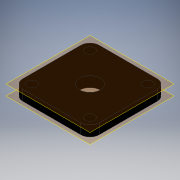
# Autodesk Inventor part: bushing
Saved by Autodesk Inventor 2016 (Build 200138000, 138)
## iProperties
Created: 2015-12-01
Part Number: bushing
Material: Generic
Document SubType Name: Modeling
Designer: Javier
Density: 1 g/cm^3
Appearance: Black
Author: Javier
Autodesk Inventor part; units mm, degrees
ref_plane "YZ Plane" through (0, 0, 0) normal (1, 0, 0) x (0, 1, 0)
ref_plane "XY Plane" through (0, 0, 0) normal (0, 0, 1) x (1, 0, 0)
sketch "Sketch1" plane through (0, 0, 0) normal (0, 1, 0) x (-1, 0, 0)
  line L0 (36.068, -47.498) -> (-36.068, -47.498)
  line L1 (-47.498, -36.068) -> (-47.498, 36.068)
  line L2 (-36.068, 47.498) -> (36.068, 47.498)
  line L3 (47.498, 36.068) -> (47.498, -36.068)
  line L4 (0, -89.5845) -> (0, 104.4956)
  line L5 (80.9625, 0) -> (-125.4125, 0)
  arc A0 (36.068, -47.498) -> (47.498, -36.068) centre (36.068, -36.068) ccw
  arc A1 (-47.498, -36.068) -> (-36.068, -47.498) centre (-36.068, -36.068) ccw
  arc A2 (47.498, 36.068) -> (36.068, 47.498) centre (36.068, 36.068) ccw
  arc A3 (-36.068, 47.498) -> (-47.498, 36.068) centre (-36.068, 36.068) ccw
  circle A4 centre (36.068, -36.068) radius 5.715
  circle A5 centre (-36.068, -36.068) radius 5.715
  circle A6 centre (36.068, 36.068) radius 5.715
  circle A7 centre (-36.068, 36.068) radius 5.715
  point P0 (0, 0)
  point P1 (47.498, -47.498)
  dimension "d0" = 94.996
  dimension "d1" = 94.996
  dimension "d2" = 11.43
  dimension "d3" = 11.43
  dimension "d4" = 11.43
  dimension "d5" = 11.43
  dimension "d6" = 11.43
  dimension "d7" = 11.43
  dimension "d8" = 11.43
  dimension "d9" = 11.43
  constraints: 12 end point, 8 centre point, 8 point on circle, 8 tangent, 4 coincident, 2 horizontal, 2 parallel, 2 point on line, 1 perpendicular, 1 vertical, 2 other
  measures "d0" distance from line of L1 point (47.498, -47.498)
  measures "d1" distance between parallel lines of L2 L0
  measures "d2" radius of A0
  measures "d3" radius of A1
  measures "d4" radius of A2
  measures "d5" radius of A3
  measures "d6" diameter of A4
  measures "d7" diameter of A5
  measures "d8" diameter of A6
  measures "d9" diameter of A7
extrude "Extrusion1" add sketch "Sketch1" along normal blind 12.954
ref_plane "Work Plane1" through (0, 12.954, 0) normal (0, 1, 0) x (-1, 0, 0)
sketch "Sketch2" plane through (0, 12.954, 0) normal (0, 1, 0) x (-1, 0, 0)
  circle A0 centre (36.068, 36.068) radius 5.715 projected
  circle A1 centre (36.068, 36.068) radius 5.715
  circle A2 centre (-36.0828, 36.068) radius 5.7002
  circle A3 centre (0, 0) radius 12.7
  dimension "d13" = 25.4
  constraints: 3 centre point, 2 coincident
  measures "d13" diameter of A3
extrude "Extrusion2" cut sketch "Sketch2" against normal blind 12.954 contours A3
body "Solid1"
